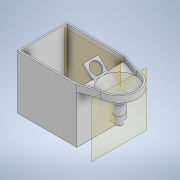
# Autodesk Inventor part: Resoar V2
Saved by Autodesk Inventor 2021 (Build 250183000, 183)
## iProperties
Created: 2025-01-08
Part Number: Resoar V2
Material: Generic
Document SubType Name: Modeling
Designer: 24lucsil
Density: 1 g/cm^3
Appearance: Default
Author: 24lucsil
Autodesk Inventor part; units mm, degrees
ref_plane "YZ Plane" through (0, 0, 0) normal (1, 0, 0) x (0, 1, 0)
ref_plane "XZ Plane" through (0, 0, 0) normal (0, 1, 0) x (-1, 0, 0)
ref_plane "XY Plane" through (0, 0, 0) normal (0, 0, 1) x (1, 0, 0)
sketch "Sketch1" plane through (0, 0, 0) normal (0, 1, 0) x (-1, 0, 0)
  line L0 (0, 0) -> (-120, 0)
  line L1 (-120, 0) -> (-120, -100)
  line L2 (-120, -100) -> (0, -100)
  line L3 (0, -100) -> (0, 0)
  dimension "d0" = 120
  dimension "d1" = 100
  constraints: 8 end point, 2 parallel, 1 horizontal, 1 perpendicular
  measures "d0" distance of L0.start L0.end
  measures "d1" distance of L2.end L0.start
extrude "Extrusion1" add sketch "Sketch1" along normal blind 3
sketch "Sketch2" plane through (0, 3, 0) normal (0, 1, 0) x (1, 0, 0)
  line L0 (0, 100) -> (0, 0) construction
  line L1 (0, 0) -> (3, 0) construction
  line L2 (3, 0) -> (3, 3) construction
  line L3 (3, 3) -> (0, 3) construction
  line L4 (0, 3) -> (0, 0) construction
  line L5 (120, 100) -> (0, 100) construction
  line L6 (120, 100) -> (117, 100) construction
  line L7 (117, 100) -> (117, 97) construction
  line L8 (117, 97) -> (120, 97) construction
  line L9 (120, 97) -> (120, 100) construction
  line L10 (3, 3) -> (117, 3)
  line L11 (117, 3) -> (117, 97)
  line L12 (117, 97) -> (3, 97)
  line L13 (3, 97) -> (3, 3)
  line L14 (120, 0) -> (120, 100) projected
  line L15 (0, 0) -> (120, 0)
  line L16 (120, 0) -> (120, 100)
  line L17 (120, 100) -> (0, 100)
  line L18 (0, 100) -> (0, 0)
  dimension "d4" = 3
  dimension "d5" = 3
  dimension "d6" = 3
  dimension "d7" = 3
  constraints: 32 end point, 8 parallel, 4 horizontal, 4 perpendicular
  measures "d4" distance of L6.end L7.end
  measures "d5" distance of L7.end L8.end
  measures "d6" distance of L2.end L3.end
  measures "d7" distance of L1.end L2.end
extrude "Extrusion2" add sketch "Sketch2" along normal blind 97
ref_plane "Work Plane1" through (155, 0, 0) normal (1, 0, 0) x (0, 0, -1)
sketch "Sketch3" plane through (155, 0, 0) normal (1, 0, 0) x (0, 0, -1)
  line L0 (0, 0) -> (0, 100) construction
  line L1 (0, 0) -> (50, 0) construction
  line L2 (100, 0) -> (0, 0) construction
  line L3 (50, 0) -> (50, 35) construction
  line L4 (50, 35) -> (43, 35) construction
  line L5 (50, 35) -> (50, 73) construction
  line L6 (50, 73) -> (40, 73) construction
  line L7 (40, 73) -> (40, 54) construction
  line L8 (43, 35) -> (40, 54)
  line L9 (40, 54) -> (40, 73)
  line L10 (3, 100) -> (97, 100) construction
  line L11 (50, 100) -> (15, 100) construction
  line L12 (15, 100) -> (15, 97)
  line L13 (15, 97) -> (40, 73)
  line L14 (15, 100) -> (43, 73)
  line L15 (43, 73) -> (43, 54)
  line L16 (43, 35) -> (45, 35)
  line L17 (43, 54) -> (45, 35)
  dimension "d11" = 35
  dimension "d12" = 7
  dimension "d13" = 38
  dimension "d14" = 10
  dimension "d15" = 35
  dimension "d16" = 3
  dimension "d81" = 19
  dimension "d82" = 3
  dimension "d83" = 2
  dimension "d84" = 19
  constraints: 30 end point, 5 vertical, 2 midpoint, 2 point on line, 1 collinear, 1 horizontal, 1 perpendicular
  measures "d11" distance of L1.end L3.end
  measures "d12" distance of L3.end L4.end
  measures "d13" distance of L3.end L5.end
  measures "d14" distance of L5.end L6.end
  measures "d15" distance of L11.end L11.start
  measures "d16" distance of L11.end L12.end
  measures "d81" distance of L6.end L7.end
  measures "d82" distance between parallel lines of L7 L15
  measures "d83" distance of L4.end L16.end
  measures "d84" vertical distance of L15.end L16.end
revolve "Revolution1" add sketch "Sketch3" angle 360 about axis through (155, 35, -50) along (0, 1, 0)
sketch "Sketch4" plane through (0, 100, 0) normal (0, 1, 0) x (1, 0, 0)
  line L0 (120, 0) -> (120, 100) projected
  line L1 (120, 0) -> (120, 3)
  line L2 (120, 100) -> (0, 100) projected
  line L3 (120, 100) -> (120, 97)
  line L4 (120, 97) -> (120, 3)
  circle A0 centre (155, 50) radius 5 projected
  circle A1 centre (155, 50) radius 35
  circle A2 centre (155, 50) radius 38
  line L5 (120, 0) -> (120, 100) projected
  line L6 (120, 0) -> (155, 12)
  line L7 (155, 88) -> (120, 100)
  point P0 (0, 0)
  point P1 (120, 50)
  dimension "d18" = 3
  dimension "d19" = 3
  dimension "d89" = 70
  dimension "d90" = 3
  constraints: 10 end point, 2 centre point, 2 coincident, 2 point on circle, 2 point on line, 1 vertical
  measures "d18" distance of L1.end L0.start
  measures "d19" distance of L0.end L3.end
  measures "d89" diameter of A1
  measures "d90" radial gap between concentric circles of A2 A1
extrude "Extrusion3" add sketch "Sketch4" against normal blind 3 contours L0 A2 L6 | A2 L0 | L0 L7 A2 picked at (191.3899, 55.4147)
sketch "Sketch5" plane through (0, 100, 0) normal (0, 1, 0) x (1, 0, 0)
  line L0 (120, 0) -> (120, 100) projected
  line L1 (0, 100) -> (0, 0) projected
  line L2 (120, 0) -> (0, 0)
  line L3 (0, 0) -> (0, 100)
  line L4 (0, 100) -> (120, 100)
  line L5 (120, 100) -> (120, 0)
  circle A0 centre (155, 50) radius 35 projected
  line L6 (117, 3) -> (117, 97) projected
  line L7 (117, 3) -> (3, 3) projected
  line L8 (3, 3) -> (3, 97) projected
  line L9 (117, 3) -> (3, 3)
  line L10 (3, 3) -> (3, 97)
  line L11 (3, 97) -> (117, 97)
  line L12 (117, 97) -> (117, 3)
  circle A1 centre (155, 50) radius 35
  circle A2 centre (155, 50) radius 38
  line L13 (0, 0) -> (120, 0) projected
  line L14 (120, 100) -> (155, 88) projected
  line L15 (120, 100) -> (155, 88)
  line L16 (155, 12) -> (120, 0) projected
  line L17 (120, 0) -> (155, 12)
  line L18 (120, 50) -> (120, 0) projected
  line L19 (120, 3) -> (155, 15)
  line L20 (120, 100) -> (120, 50) projected
  line L21 (120, 97) -> (155, 85)
  line L22 (155, 88) -> (120, 100) projected
  line L23 (117, 3) -> (120, 3)
  line L24 (120, 97) -> (117, 97)
  dimension "d85" = 3
  dimension "d91" = 37
  dimension "d92" = 37
  constraints: 28 end point, 8 equal length, 2 centre point, 2 coincident, 2 horizontal, 2 perpendicular, 2 point on circle, 2 point on line, 1 concentric
  measures "d85" radial gap between concentric circles of A2 A0
  measures "d91" distance of L19.start L19.end
  measures "d92" distance of L21.start L21.end
extrude "Extrusion4" add sketch "Sketch5" along normal blind 10 contours L2 L1 L4 L0 L24 L11 L8 L7 L23 | L0 L19 A2 L16 | A2 L19 A0 L21 | L14 A2 L21 L0
ref_plane "Work Plane2" through (3, 3, -65) normal (0, 0, 1) x (1, 0, 0)
sketch "Sketch6" plane through (3, 3, -65) normal (0, 0, 1) x (1, 0, 0)
  line L0 (0, 0) -> (0, 107) projected
  line L1 (0, 0) -> (0, 21.21)
  line L2 (0, 0) -> (114, 0) projected
  line L3 (0, 0) -> (21.21, 0)
  line L4 (114, 0) -> (0, 0) projected
  line L5 (0, 21.21) -> (21.21, 0)
  line L6 (0, 21.21) -> (0, 17.21)
  line L7 (0, 17.21) -> (17.21, 0)
  point P0 (-3, -3)
  point P1 (0, 17.21)
  point P2 (17.21, 0)
  point P3 (21.21, 0)
  point P4 (0, 97)
  dimension "d26" = 21.21
  dimension "d27" = 21.21
  dimension "d28" = 4
  constraints: 10 end point, 4 point on line, 1 parallel
  measures "d26" distance from line of L2 L1.end
  measures "d27" distance of L0.start L3.end
  measures "d28" distance of L6.end L1.end
extrude "Extrusion5" add sketch "Sketch6" along normal blind 30 contours L0 L5 L2 L7
sketch "Sketch7" plane through (3, 24.21, -65) normal (0.7071, 0.7071, 0) x (-0.7071, 0.7071, 0)
  line L0 (-29.9955, 30) -> (0, 30) projected
  line L1 (-14.9977, 30) -> (-14.9977, 15)
  circle A0 centre (-14.9977, 15) radius 11.5
  point P0 (-14.9977, 65)
  dimension "d31" = 15
  dimension "d32" = 23
  constraints: 2 end point, 1 centre point, 1 coincident, 1 midpoint, 1 vertical
  measures "d31" distance of L1.start L1.end
  measures "d32" diameter of A0
extrude "Extrusion6" cut sketch "Sketch7" against normal blind 3.6
sketch "Sketch11" plane through (3, 3, -65) normal (0, 0, 1) x (1, 0, 0)
  line L0 (18.7367, 2.4733) -> (16.7367, 0.4733) construction
  line L1 (18.7367, 2.4733) -> (148.7367, 132.4733) construction
  line L2 (2.4733, 18.7367) -> (0.4733, 16.7367) construction
  line L3 (2.4733, 18.7367) -> (132.4733, 148.7367) construction
  line L4 (113.7569, 97.4935) -> (95.3721, 115.8782) construction
  line L5 (95.3721, 115.8782) -> (92.3721, 112.8782) construction
  line L6 (92.3721, 112.8782) -> (113.7569, 91.4935) construction
  line L7 (117, 97) -> (145, 70) projected
  line L8 (117, 97) -> (113.4034, 97.847)
  line L9 (113.4034, 97.847) -> (95.3721, 115.8782)
  line L10 (95.3721, 115.8782) -> (92.3721, 112.8782)
  line L11 (92.3721, 112.8782) -> (110.7569, 94.4935)
  line L12 (110.7569, 94.4935) -> (114, 85.7766)
  line L13 (114, 0) -> (114, 97) projected
  line L14 (114, 85.7766) -> (117, 85.7766)
  line L15 (117, 85.7766) -> (117, 97)
  line L16 (117, 94) -> (117, 107) projected
  point P0 (-3, -3)
  dimension "d65" = 130
  dimension "d66" = 130
  dimension "d67" = 26
  dimension "d68" = 3
  dimension "d69" = 134.3788
  dimension "d70" = 4.2426
  dimension "d71" = 49.4689
  dimension "d72" = 49.4689
  dimension "d73" = 25.634
  dimension "d74" = 149.293
  dimension "d75" = 0
  constraints: 24 end point, 7 point on line, 4 collinear, 3 perpendicular, 2 parallel
  measures "d65" horizontal distance of L3.start L3.end
  measures "d66" horizontal distance of L1.start L1.end
  measures "d67" distance of L4.start L4.end
  measures "d68" horizontal distance of L4.end L5.end
  measures "d69" distance from line of L0.start L4
  measures "d70" distance from line of L6.end L0
  measures "d71" distance from line of L1.end L4
  measures "d72" distance from line of L3.end L4
  measures "d73" angle of L7 L12
  measures "d74" angle of L8 L7
  measures "d75" distance between parallel lines of L15 L16
extrude "Extrusion8" add sketch "Sketch11" along normal blind 30
sketch "Sketch12" plane through (3, 24.21, -65) normal (0.7071, 0.7071, 0) x (-0.7071, 0.7071, 0)
  line L0 (-14.9977, -32) -> (-14.9977, 62) projected
  circle A0 centre (-14.9977, 15) radius 11.5
  point P0 (-14.9977, 65)
  dimension "d78" = 23
  constraints: 1 centre point, 1 midpoint
  measures "d78" diameter of A0
extrude "Extrusion9" cut sketch "Sketch12" along normal through all
body "Solid1"
